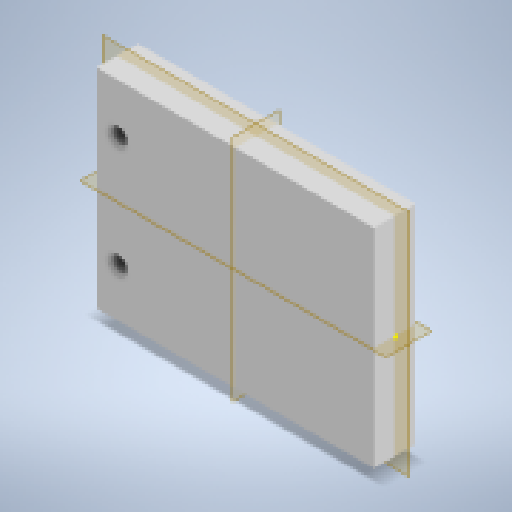
# Autodesk Inventor part: крыло
Saved by Autodesk Inventor 2023.2 (Build 272271030, 271C)
## iProperties
Created: 2024-03-20
Part Number: крыло
Material: Типовые
Document SubType Name: Modeling
Designer: I9232
Density: 1 g/cm^3
Appearance: По умолчанию
Author: I9232
Autodesk Inventor part; units mm, degrees
sketch "Эскиз1" plane through (0, 0, 0) normal (0, 0, 1) x (1, 0, 0)
  line L0 (-20, -15) -> (20, -15)
  line L1 (20, -15) -> (20, 15)
  line L2 (20, 15) -> (-20, 15)
  line L3 (-20, 15) -> (-20, -15)
  line L4 (-20, -15) -> (20, 15) construction
  line L5 (20, -15) -> (-20, 15) construction
  point P0 (0, 0)
  dimension "d0" = 40
  dimension "d1" = 30
  constraints: 12 end point, 2 midpoint, 2 parallel, 1 horizontal, 1 perpendicular
  measures "d0" distance of L1.end L2.end
  measures "d1" distance of L0.end L1.end
extrude "Выдавливание1" add sketch "Эскиз1" along normal mid plane 6
sketch "Эскиз2" plane through (0, 0, -3) normal (0, 0, -1) x (-1, 0, 0)
  circle A0 centre (16.75, 8) radius 1.25 projected
  circle A1 centre (16.75, -8) radius 1.25 projected
  point P0 (0, 0)
extrude "Выдавливание2" cut sketch "Эскиз2" against normal up to surface (6 mm away)
sketch "Эскиз3" plane through (20, -15, 3) normal (1, 0, 0) x (0, 0, -1)
  line L0 (0, 0) -> (0, 30) projected
  line L1 (6, 0) -> (6, 30) projected
  line L2 (0, 0) -> (6, 0)
  line L3 (6, 0) -> (6, 5)
  line L4 (6, 5) -> (0, 5)
  line L5 (0, 5) -> (0, 0)
  line L6 (0, 25) -> (6, 25)
  line L7 (6, 25) -> (6, 30)
  line L8 (6, 30) -> (0, 30)
  line L9 (0, 30) -> (0, 25)
  line L10 (6, 30) -> (6, 0) projected
  line L11 (0, 10) -> (6, 10)
  line L12 (6, 10) -> (6, 15)
  line L13 (0, 15) -> (0, 10)
  line L14 (0, 20) -> (6, 20)
  line L15 (6, 20) -> (6, 15)
  line L16 (0, 15) -> (0, 20)
  point P0 (3, 15)
  point P1 (0, 5)
  point P2 (0, 25)
  point P3 (6, 25)
  point P4 (6, 10)
  dimension "d6" = 5
  dimension "d7" = 5
  dimension "d20" = 5
  dimension "d22" = 5
  constraints: 28 end point, 6 parallel, 5 point on line, 4 horizontal, 4 perpendicular, 2 midpoint
  measures "d6" distance of L0.end L6.start
  measures "d7" distance of L4.end L0.start
  measures "d20" distance between parallel lines of L4 L11
  measures "d22" distance between parallel lines of L14 L6
extrude "Выдавливание3" add sketch "Эскиз3" along normal blind 3 contours L0 L4 L1 L2 | L0 L14 L1 L11 | L0 L8 L1 L6
sketch "Эскиз4" plane through (0, 0, 3) normal (0, 0, 1) x (1, 0, 0)
  line L0 (20, 6.05) -> (20, 8.95)
  line L1 (4.1, 8.95) -> (4.1, 6.05)
  line L2 (10.1, 10.3) -> (11.9, 10.3)
  line L3 (11.9, 4.7) -> (10.1, 4.7)
  line L4 (20, 8.95) -> (11.9, 8.95)
  line L5 (10.1, 8.95) -> (4.1, 8.95)
  line L6 (10.1, 4.7) -> (10.1, 6.05)
  line L7 (10.1, 8.95) -> (10.1, 10.3)
  line L8 (11.9, 10.3) -> (11.9, 8.95)
  line L9 (11.9, 6.05) -> (11.9, 4.7)
  line L10 (4.1, 6.05) -> (10.1, 6.05)
  line L11 (11.9, 6.05) -> (20, 6.05)
  line L12 (20, 5) -> (20, 10) projected
  line L13 (1.3154, 0) -> (2.8284, 0) construction
  line L14 (20, -6.05) -> (20, -8.95)
  line L15 (4.1, -8.95) -> (4.1, -6.05)
  line L16 (10.1, -10.3) -> (11.9, -10.3)
  line L17 (11.9, -4.7) -> (10.1, -4.7)
  line L18 (20, -8.95) -> (11.9, -8.95)
  line L19 (10.1, -8.95) -> (4.1, -8.95)
  line L20 (10.1, -4.7) -> (10.1, -6.05)
  line L21 (10.1, -8.95) -> (10.1, -10.3)
  line L22 (11.9, -10.3) -> (11.9, -8.95)
  line L23 (11.9, -6.05) -> (11.9, -4.7)
  line L24 (4.1, -6.05) -> (10.1, -6.05)
  line L25 (11.9, -6.05) -> (20, -6.05)
  point P0 (0, 0)
  point P1 (20, 0)
  point P2 (20, 7.5)
  dimension "d10" = 2.9
  dimension "d11" = 1.8
  dimension "d12" = 5.6
  dimension "d14" = 1.35
  dimension "d15" = 6
  dimension "d16" = 8.1
  constraints: 50 end point, 12 symmetric about line, 10 parallel, 4 equal length, 4 horizontal, 4 perpendicular, 2 midpoint, 1 point on line
  measures "d10" distance of L0.start L0.end
  measures "d11" distance of L2.start L2.end
  measures "d12" distance of L2.end L3.start
  measures "d14" distance of L5.start L2.start
  measures "d15" distance of L5.start L1.start
  measures "d16" distance of L0.end L4.end
extrude "Выдавливание4" cut sketch "Эскиз4" against normal up to surface (6 mm away)
sketch "Эскиз5" plane through (0, 0, 3) normal (0, 0, 1) x (1, 0, 0)
  line L0 (-6, 2) -> (-10, 2) projected
  line L1 (-10, 2) -> (-10, -2) projected
  line L2 (-10, -2) -> (-6, -2) projected
  line L3 (-6, -2) -> (-6, 2) projected
  line L4 (-1, 2) -> (-1, -2) projected
  line L5 (-1, -2) -> (3, -2) projected
  line L6 (3, -2) -> (3, 2) projected
  line L7 (3, 2) -> (-1, 2) projected
  line L8 (7, 2) -> (7, -2) projected
  line L9 (11, 2) -> (7, 2) projected
  line L10 (7, -2) -> (11, -2) projected
  line L11 (11, -2) -> (11, 2) projected
  line L12 (16, 2) -> (16, -2) projected
  line L13 (20, 2) -> (16, 2) projected
  line L14 (16, -2) -> (20, -2) projected
  line L15 (20, -2) -> (20, 2) projected
  point P0 (0, 0)
extrude "Выдавливание5" cut sketch "Эскиз5" against normal up to surface (6 mm away)
sketch "Эскиз6" plane through (0, 0, 3) normal (0, 0, 1) x (1, 0, 0)
  circle A0 centre (-3.5, 0) radius 1.5
  circle A1 centre (13.5, 0) radius 1.5
  line L0 (-6, 2) -> (-6, -2) projected
  line L1 (-1, -2) -> (-1, 2) projected
  line L2 (11, 2) -> (11, -2) projected
  line L3 (16, -2) -> (16, 2) projected
  line L4 (-6, 0) -> (-1, 0) construction
  line L5 (11, 0) -> (16, 0) construction
  point P0 (0, 0)
  point P1 (-3.5, 0)
  point P2 (13.5, 0)
  dimension "d25" = 3
  constraints: 6 midpoint, 4 end point, 2 centre point, 2 coincident, 1 equal radius
  measures "d25" diameter of A0
extrude "Выдавливание6" cut sketch "Эскиз6" against normal up to surface (6 mm away)
